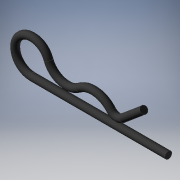
# Autodesk Inventor part: RNPN10
Saved by Autodesk Inventor 2019 (Build 230136000, 136)
## iProperties
Created: 2023-01-18
Part Number: RNPN10
Material: Generic
Catalog Web Link: www.cadenas.de
Description: RNPN-Hair Pins
Vendor: MISUMI
Document SubType Name: Modeling
Designer: psAdmin
Manufacturer: MISUMI
Mass: 0.211807 g
Surface Area: 4.75798 cm^2
Volume: 0.211807 cm^3
Density: 1 g/cm^3
Appearance: PSOLRGB-175-175-175
Category: PARTsolutions
Company: MISUMI
Title: RNPN10
Author: Cadenas PARTsolutions
Comments: Hair Pins
PSOL_IDENT_0: {$CADENAS_DATA/23d-libs/misumi/metric/28_keys_magnets/rnpn.prj},150 {VTYP=3D},{NB=RNPN10},{LINA=RNPN
PSOL_IDENT_1: 10},{NN=RNPN},{DATE=30.06.2021 13:10:00},{GEOMDATE=08.10.2020 09:18:12},{VERSION=},{LINEID=30},{WBVA
PSOL_IDENT_2: R=},{WBNUMERIC=}  {NB=RNPN10},{LINA=RNPN10},{KT=DUMMY},{PN=RNPN10},{TS=RNPN},{MAT=JIS-SWRH6},{ST=Tri
PSOL_IDENT_3: valent Chromate Plating},{NO=10},{DD=1.8},{L=40.2},{L1=15.7},{L2=5.7},{R=5},{HH=3.0},{D1=10},{D2=2.2
PSOL_IDENT_4: },{ANG1=37.9},{ANG2=50.5},{ANG3=108.4},{ANG4=19.5},{ANG5=90.5},{CU1=6.0},{CU2=3.0},{CU3=3.5},{LE1=7.
PSOL_IDENT_5: 0478}
NB: RNPN10
NN: RNPN
NT: Hair Pins
NBSYN: $PN.
LINA: RNPN10
CATALOG: Misumi
PN: RNPN10
MAT: JIS-SWRH6
ST: Trivalent Chromate Plating
NO: 10
DD: 1.8
L: 40.2
L1: 15.7
L2: 5.7
R: 5
HH: 3
D1: 10
D2: 2.2
SUPPLIER: MISUMI
ARTICLENO: RNPN10
BOMINFO: RNPN10
CREATOR: CADENAS GmbH
Autodesk Inventor part; units mm, degrees
sketch "Sketch_2" plane through (-0.6757, -0.232, 0) normal (0.7890841, 0.6142852, 0) x (0, 0, -1)
  line L0 (10, -1.1) -> (-10, -1.1)
  circle A0 centre (0, 4.8) radius 0.9
  constraints: 2 end point, 1 centre point
revolve "Revolution1" add sketch "Sketch_2" angle 88.4 about axis through (0, -1.1, -10) along (0, 0, -1)
sketch "Sketch_3" plane through (-3.6243, 3.5556, 0) normal (-0.7890841, -0.6142852, 0) x (0, 0, 1)
  line L0 (-10, 5.1) -> (10, 5.1)
  circle A0 centre (0, 0) radius 0.9
  constraints: 2 end point, 1 centre point
revolve "Revolution2" add sketch "Sketch_3" angle 108.4 about axis through (-6.7571, 7.5799, -10) along (0, 0, -1)
sketch "Sketch_4" plane through (4.5526, 2.6529, 0) normal (0.6360782, -0.7716246, 0) x (0, 0, -1)
  line L0 (-10, 2.1) -> (10, 2.1)
  circle A0 centre (0, 0) radius 0.9
  constraints: 2 end point, 1 centre point
revolve "Revolution3" add sketch "Sketch_4" angle 90.5 about axis through (6.173, 3.9886, 10) along (0, 0, 1)
sketch "_____1" plane through (-15.7, 20.1, 0) normal (-1, 0, 0) x (0, 1, 0)
  line L0 (-15.7, 10) -> (-15.7, -10)
  circle A0 centre (-20.1, 0) radius 0.9
  constraints: 2 end point, 1 centre point
revolve "Revolution4" add sketch "_____1" angle 250.5 about axis through (-15.7, 4.4, -10) along (0, 0, -1)
sketch "Sketch_7" plane through (0, 0, 0) normal (0, 0, 1) x (1, 0, 0)
  line L0 (-15.7, 0) -> (19.2, 0)
  line L1 (19.2, 0) -> (19.2, -0.9)
  line L2 (19.2, -0.9) -> (-15.7, -0.9)
  line L3 (-15.7, -0.9) -> (-15.7, 0)
  line L4 (-15.7, 0) -> (19.2, 0)
  constraints: 10 end point
revolve "Revolution5" add sketch "Sketch_7" angle 360 about axis through (-15.7, 0, 0) along (-1, 0, 0)
sketch "_____2" plane through (7.5229, 2.3799, 0) normal (0.7660444, 0.6427876, 0) x (0, 0, -1)
  circle A0 centre (0, 0) radius 0.9
  constraints: 1 centre point
extrude "Extrusion1" add sketch "_____2" along normal blind 7.0478
ref_plane "c1_XY" through (0, 0, 0) normal (1, 0, 0) x (0, 0, -1)
ref_plane "c1_YZ" through (0, 0, 0) normal (0, 0, -1) x (0, 1, 0)
ref_plane "c1_ZX" through (0, 0, 0) normal (0, 1, 0) x (1, 0, 0)
ref_plane "to_sahft_XY" through (0, 0, 0) normal (0, 0, 1) x (1, 0, 0)
ref_plane "to_sahft_YZ" through (0, 0, 0) normal (1, 0, 0) x (0, 1, 0)
ref_plane "to_sahft_ZX" through (0, 0, 0) normal (0, 1, 0) x (0, 0, 1)
body "Solid1"
